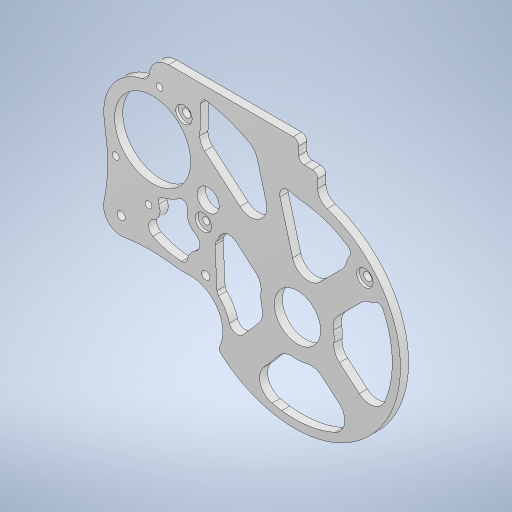
# Autodesk Inventor part: 足内フレーム
Saved by Autodesk Inventor 2023 (Build 270158000, 158)
## iProperties
Created: 2022-01-10
Part Number: 足内フレーム
Material: Aluminum 2014-T4
Document SubType Name: Modeling
Designer: acps
Density: 2.8 g/cm^3
Appearance: Satin
Author: acps
Autodesk Inventor part; units mm, degrees
ref_plane "YZ Plane" through (0, 0, 0) normal (1, 0, 0) x (0, 1, 0)
ref_plane "XZ Plane" through (0, 0, 0) normal (0, 1, 0) x (-1, 0, 0)
ref_plane "XY Plane" through (0, 0, 0) normal (0, 0, 1) x (1, 0, 0)
sketch "Sketch9" plane through (0, 0, 0) normal (0, 0, 1) x (1, 0, 0)
  circle A0 centre (46.616, 30) radius 14
  circle A1 centre (67.0906, 21) radius 20.5 construction
  arc A2 (93.8028, -35.6609) -> (110.9454, 40.1044) centre (98.9344, 3) ccw
  arc A3 (28.8684, 26.9964) -> (93.8028, -35.6609) centre (103.8028, 39.6783) ccw construction
  arc A4 (71.3782, -23.4684) -> (59.8142, -6.4542) centre (60.4847, -18.4355) ccw
  arc A5 (71.3782, -23.4684) -> (71.8871, -25.8212) centre (73.1938, -24.3072) ccw
  arc A6 (71.8871, -25.8212) -> (93.8028, -35.6609) centre (99.3292, 5.9739) ccw
  circle A7 centre (65.359, 13) radius 3
  circle A8 centre (66.1789, -3.483) radius 4 construction
  circle A9 centre (66.1789, -3.483) radius 3
  circle A10 centre (66.1789, -3.483) radius 1.5
  circle A11 centre (49.1519, 48.073) radius 1.25
  circle A12 centre (45.1, 8.5) radius 1.25
  circle A13 centre (33, 18) radius 1.25
  arc A14 (119.1717, 29.0833) -> (128.6406, 19.1104) centre (124.8574, 25) ccw
  arc A15 (131.5325, 18.2763) -> (128.6406, 19.1104) centre (129.7215, 17.4276) ccw
  arc A16 (119.1717, 29.0833) -> (118.6753, 31.9015) centre (117.5473, 30.25) ccw
  circle A17 centre (67.0906, 21) radius 1.5
  circle A18 centre (67.0906, 21) radius 4.5 construction
  circle A19 centre (49.1519, 48.073) radius 4.25 construction
  arc A20 (42.888, 47.6097) -> (45.3636, 50.3845) centre (42.2376, 50.6816) ccw
  arc A21 (42.888, 47.6097) -> (28.8684, 26.9964) centre (46.616, 30) ccw
  arc A22 (52.4852, 56.8614) -> (45.3636, 50.3845) centre (52.4852, 49.7076) ccw
  arc A23 (118.6753, 31.9015) -> (102.5834, 37.8093) centre (98.9344, 3) ccw
  arc A24 (88.285, 43.2258) -> (102.5834, 37.8093) centre (105.7111, 67.6458) ccw
  arc A25 (88.285, 43.2258) -> (66.7822, 52.3614) centre (56.9182, -0.7301) ccw
  arc A26 (66.7822, 52.3614) -> (64.4184, 50.4721) centre (66.4169, 50.395) ccw
  line L0 (64.4184, 50.4721) -> (63.6467, 30.4665)
  arc A27 (63.6467, 30.4665) -> (65.9495, 28.4127) centre (65.6452, 30.3894) ccw
  arc A28 (72.0057, 15.3351) -> (65.9495, 28.4127) centre (67.0906, 21) ccw
  arc A29 (62.3527, 39.5241) -> (63.2626, 46.965) centre (58.1571, 43.8132) ccw construction
  arc A30 (72.0057, 15.3351) -> (71.327, 13.6183) centre (73.3164, 13.8244) ccw
  arc A31 (70.0506, 9.2598) -> (71.327, 13.6183) centre (65.359, 13) ccw
  arc A32 (63.4085, 27.3516) -> (62.8815, 34.943) centre (46.616, 30) ccw construction
  arc A33 (70.0506, 9.2598) -> (69.6169, 7.9138) centre (71.6145, 8.0131) ccw
  line L1 (69.6169, 7.9138) -> (70.3257, -6.3345)
  arc A34 (70.3257, -6.3345) -> (70.9304, -7.6704) centre (72.3232, -6.2351) ccw
  arc A35 (74.8454, -22.768) -> (70.9304, -7.6704) centre (60.4847, -18.4355) ccw
  arc A36 (75.5402, -24.9305) -> (94.1976, -32.687) centre (99.3292, 5.9739) ccw
  arc A37 (74.8454, -22.768) -> (75.5402, -24.9305) centre (76.7601, -23.3457) ccw
  line L2 (65.359, 13) -> (66.1789, -3.483) construction
  arc A38 (94.1976, -32.687) -> (131.5325, 18.2763) centre (98.9344, 3) ccw
  arc A39 (29.8929, 18.5469) -> (54.2095, -6.2157) centre (58.2196, 22.0427) ccw
  arc A40 (50.2005, 13.3822) -> (56.3412, 16.0565) centre (46.616, 30) ccw
  arc A41 (59.4537, 14.062) -> (56.3412, 16.0565) centre (57.4853, 14.4161) ccw
  arc A42 (46.8589, 4.6311) -> (48.8551, 10.4905) centre (45.1, 8.5) ccw
  arc A43 (59.4537, 14.062) -> (62.4846, 7.7333) centre (65.359, 13) ccw
  arc A44 (46.7538, -0.7807) -> (57.3342, -3.4835) centre (58.2196, 22.0427) ccw
  arc A45 (62.5868, 2.5251) -> (59.3536, -1.9287) centre (66.1789, -3.483) ccw
  arc A46 (57.3342, -3.4835) -> (59.3536, -1.9287) centre (57.4035, -1.4847) ccw
  arc A47 (50.2005, 13.3822) -> (48.8551, 10.4905) centre (50.6222, 11.4271) ccw
  arc A48 (62.5868, 2.5251) -> (62.4846, 7.7333) centre (61.0474, 5.1) ccw
  arc A49 (46.8589, 4.6311) -> (46.7538, -0.7807) centre (48.1006, 1.9001) ccw
  circle A50 centre (33, 18) radius 3 construction
  line L3 (29.8929, 18.5469) -> (28.7516, 27.7953)
  circle A51 centre (124.8574, 25) radius 3
  circle A52 centre (124.8574, 25) radius 1.5
  circle A53 centre (100, 0) radius 6.025 construction
  circle A54 centre (100, 0) radius 30 construction
  circle A55 centre (100, 0) radius 8.525
  circle A56 centre (100, 0) radius 13.525
  circle A57 centre (58.1571, 43.8132) radius 3
  circle A58 centre (58.1571, 43.8132) radius 1.5
  arc A59 (116.4268, 23.6124) -> (118.0268, 26.5308) centre (112.172, 27.8429) ccw
  line L4 (116.4268, 23.6124) -> (108.2597, 15.3984)
  arc A60 (126.4272, 18.1783) -> (123.5181, 16.5616) centre (127.7728, 12.3311) ccw
  arc A61 (114.9197, 7.9139) -> (113.2822, 2.5515) centre (119.1744, 3.6834) ccw
  line L5 (114.9197, 7.9139) -> (123.5181, 16.5616)
  line L6 (100, 0) -> (74.542, 21.8523) construction
  arc A62 (91.0161, 14.3009) -> (96.4839, 13.06) centre (94.924, 18.8536) ccw
  arc A63 (86.558, 1.4963) -> (84.5028, 6.7129) centre (80.5949, 2.1601) ccw
  line L7 (77.423, 12.7899) -> (84.5028, 6.7129)
  line L8 (91.0161, 14.3009) -> (65.753, 35.9858)
  arc A64 (77.423, 12.7899) -> (71.0342, 11.0528) centre (74.8177, 9.7547) ccw
  arc A65 (64.0134, 39.9725) -> (65.753, 35.9858) centre (69.0097, 39.7797) ccw
  arc A66 (108.9839, -14.3009) -> (103.5161, -13.06) centre (105.076, -18.8536) ccw
  arc A67 (113.442, -1.4963) -> (115.4972, -6.7129) centre (119.4051, -2.1601) ccw
  line L9 (100, 0) -> (122.764, -19.5398) construction
  line L10 (108.9839, -14.3009) -> (115.3122, -19.7328)
  line L11 (115.4972, -6.7129) -> (122.7736, -12.9587)
  arc A68 (113.8982, -29.7427) -> (115.3122, -19.7328) centre (111.4042, -24.2856) ccw
  arc A69 (122.7736, -12.9587) -> (132.231, -10.6871) centre (126.6816, -8.4059) ccw
  arc A70 (85.6991, -8.9839) -> (86.94, -3.5161) centre (81.1464, -5.076) ccw
  arc A71 (98.5037, -13.442) -> (93.2871, -15.4972) centre (97.8399, -19.4051) ccw
  line L12 (85.6991, -8.9839) -> (80.0896, -15.5191)
  line L13 (87.4521, -22.2951) -> (93.2871, -15.4972)
  arc A72 (74.9251, -14.3768) -> (80.0896, -15.5191) centre (77.8132, -13.5651) ccw
  arc A73 (87.4521, -22.2951) -> (90.6732, -32.0534) centre (92.0049, -26.203) ccw
  circle A74 centre (67.0906, 21) radius 4.025
  arc A75 (78.8207, 24.7689) -> (88.5197, 30.8912) centre (82.7286, 29.3217) ccw
  arc A76 (85.1671, 43.2617) -> (82.1833, 46.995) centre (79.376, 41.6922) ccw
  arc A77 (97.3091, 38.8464) -> (93.5734, 35.1817) centre (96.4689, 35.9664) ccw
  line L14 (85.1671, 43.2617) -> (88.5197, 30.8912)
  line L15 (93.5734, 35.1817) -> (98.2138, 18.0594)
  circle A78 centre (35, 0) radius 1.5
  circle A79 centre (35, 0) radius 6.5
  arc A80 (28.6494, 1.3855) -> (29.7909, 19.5065) centre (-29.9717, 14.1749) ccw
  arc A81 (54.2095, -6.2157) -> (36.0536, -6.414) centre (45.7794, -65.6205) ccw
  arc A82 (54.2095, -6.2157) -> (59.8142, -6.4542) centre (58.2196, 22.0427) ccw
  line L16 (52.4852, 56.8614) -> (98.4852, 56.8614)
  arc A83 (100.4852, 54.8614) -> (98.4852, 56.8614) centre (98.4852, 54.8614) ccw
  line L17 (100.4852, 54.8614) -> (100.4852, 51.8614)
  arc A84 (100.4852, 51.8614) -> (102.4852, 49.8614) centre (102.4852, 51.8614) ccw
  line L18 (102.4852, 49.8614) -> (105.4852, 49.8614)
  arc A85 (107.4852, 47.8614) -> (105.4852, 49.8614) centre (105.4852, 47.8614) ccw
  line L19 (107.4852, 47.8614) -> (107.4852, 44.8614)
  arc A86 (107.4852, 44.8614) -> (110.9454, 40.1044) centre (112.4852, 44.8614) ccw
  line L20 (100, 0) -> (124.8574, 25) construction
  line L21 (100, 0) -> (88.285, 43.2258) construction
  arc A87 (98.2138, 18.0594) -> (108.2597, 15.3984) centre (104.0049, 19.6289) ccw
  line L22 (69.6707, 28.6693) -> (73.6138, 25.2847) construction
  line L23 (100, 0) -> (77.4284, -26.2961) construction
  circle A88 centre (65.359, 13) radius 1.25
  point P0 (0, 0)
  point P1 (100.4852, 53.3614)
  point P2 (107.4852, 46.3614)
  point P3 (65.7689, 4.7585)
  point P4 (29.8281, 19.0723)
  dimension "d389" = 2
  dimension "d390" = 42
  dimension "d391" = 74
  dimension "d392" = 118
  dimension "d393" = 6
  dimension "d394" = 8
  dimension "d395" = 6
  dimension "d396" = 3
  dimension "d397" = 2.5
  dimension "d398" = 2.5
  dimension "d399" = 8.5
  dimension "d400" = 45.1
  dimension "d401" = 2.5
  dimension "d402" = 18
  dimension "d403" = 33
  dimension "d404" = 2
  dimension "d405" = 2
  dimension "d406" = 3
  dimension "d407" = 3
  dimension "d408" = 3
  dimension "d409" = 4
  dimension "d410" = 2
  dimension "d411" = 2
  dimension "d412" = 3
  dimension "d413" = 2
  dimension "d414" = 3
  dimension "d415" = 3
  dimension "d416" = 2
  dimension "d417" = 2
  dimension "d418" = 3
  dimension "d419" = 2
  dimension "d420" = 3
  dimension "d421" = 12
  dimension "d422" = 3
  dimension "d423" = 2
  dimension "d424" = 3
  dimension "d425" = 3
  dimension "d426" = 3
  dimension "d427" = 3
  dimension "d428" = 2
  dimension "d429" = 3
  dimension "d430" = 3
  dimension "d431" = 2
  dimension "d432" = 6
  dimension "d433" = 4
  dimension "d434" = 17.05
  dimension "d435" = 5
  dimension "d436" = 3
  dimension "d437" = 6
  dimension "d438" = 6
  dimension "d439" = 6
  dimension "d440" = 6
  dimension "d441" = 6
  dimension "d442" = 10
  dimension "d443" = 5
  dimension "d444" = 4
  dimension "d445" = 5
  dimension "d446" = 6
  dimension "d447" = 6
  dimension "d448" = 10
  dimension "d449" = 5
  dimension "d450" = 6
  dimension "d451" = 6
  dimension "d452" = 6
  constraints: 143 point on circle, 87 centre point, 79 tangent, 48 end point, 12 parallel, 11 concentric, 10 coincident, 3 midpoint, 2 horizontal, 2 perpendicular, 2 point on line, 2 vertical, 1 horizontal alignment, 45 other
  measures "d389" radius of A5
  measures "d390" radius of A6
  measures "d393" diameter of A7
  measures "d394" diameter of A8
  measures "d395" diameter of A9
  measures "d396" diameter of A10
  measures "d397" diameter of A11
  measures "d398" diameter of A12
  measures "d399" vertical distance of point (0, 0) A12.centre
  measures "d400" horizontal distance of point (0, 0) A12.centre
  measures "d401" diameter of A13
  measures "d402" vertical distance of point (0, 0) A13.centre
  measures "d403" horizontal distance of point (0, 0) A13.centre
  measures "d404" radius of A15
  measures "d405" radius of A16
  measures "d406" diameter of A17
  measures "d407" radial gap between concentric circles of A17 A18
  measures "d408" radial gap between concentric circles of A11 A19
  measures "d409" radial gap between concentric circles of A23 A2
  measures "d410" radius of A26
  measures "d411" radius of A27
  measures "d412" radial gap between concentric circles of A18 A28
  measures "d413" radius of A30
  measures "d414" radial gap between concentric circles of A7 A31
  measures "d415" radial gap between concentric circles of A0 A32
  measures "d416" radius of A33
  measures "d417" radius of A34
  measures "d418" radial gap between concentric circles of A4 A35
  measures "d419" radius of A37
  measures "d420" radial gap between concentric circles of A2 A38
  measures "d421" radius of A4
  measures "d422" radial gap between concentric circles of A0 A40
  measures "d423" radius of A41
  measures "d424" radial gap between concentric circles of A12 A42
  measures "d425" radial gap between concentric circles of A7 A43
  measures "d426" radial gap between concentric circles of A39 A44
  measures "d427" radial gap between concentric circles of A45 A8
  measures "d428" radius of A47
  measures "d429" radius of A48
  measures "d430" radius of A49
  measures "d431" radius of A46
  measures "d432" diameter of A50
  measures "d433" radial gap between concentric circles of A14 A51
  measures "d434" diameter of A55
  measures "d436" radial gap between concentric circles of A29 A57
  measures "d437" radius of A59
  measures "d438" radius of A60
  measures "d439" radius of A61
  measures "d440" radius of A62
  measures "d441" radius of A63
  measures "d442" distance between parallel lines of L7 L8
  measures "d443" distance between parallel lines of L8 L6
  measures "d444" radius of A64
  measures "d445" radius of A65
  measures "d446" radius of A66
  measures "d447" radius of A67
  measures "d448" distance between parallel lines of L10 L11
  measures "d449" distance between parallel lines of L11 L9
  measures "d450" radius of A68
  measures "d451" radius of A69
  measures "d452" radius of A70
extrude "Extrusion8" add sketch "Sketch9" against normal blind 3 contours A6 A5 A4 A82 A39 A79 L3 A21 A20 A22 L16 A83 L17 A84 L18 A85 L19 A86 A2 | A81 A79 A39 | A79 A39 | A39 A79 | A79 A80 L3 A39 | A7 | A9 | A14 A60 L5 A61 A56 A62 L8 A75 L14 A76 A25 A24 A77 L15 A87 L4 A59 | A38 A68 L10 A66 A56 A67 L11 A69 | A56 | A56 A63 L7 A64 A31 A30 A28 A27 L0 A65 L8 A62 | A36 A37 A35 A72 L12 A70 A56 A71 L13 A73 | A51 | A57
extrude "Extrusion9" cut sketch "Sketch9" against normal blind 1 contours A7 | A51 | A57
body "Solid3"
